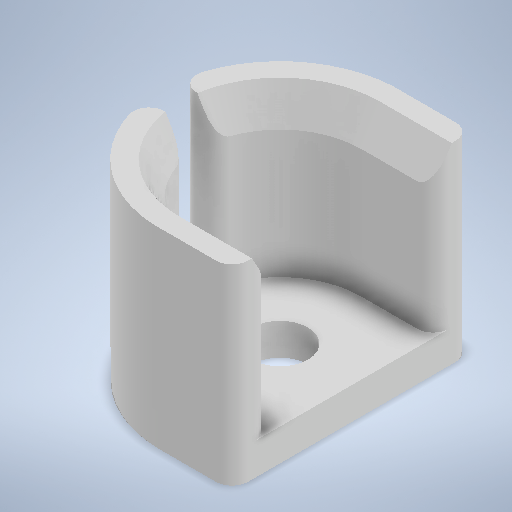
# Autodesk Inventor part: Align_Bracket
Saved by Autodesk Inventor 2025.1 (Build 291241000, 241)
## iProperties
Created: 2026-04-27
Part Number: Align_Bracket
Material: Generic
Document SubType Name: Modeling
Designer: ryand
Density: 1 g/cm^3
Appearance: Default
Author: ryand
Autodesk Inventor part; units mm, degrees
ref_plane "YZ Plane" through (0, 0, 0) normal (1, 0, 0) x (0, 1, 0)
ref_plane "XZ Plane" through (0, 0, 0) normal (0, 1, 0) x (-1, 0, 0)
ref_plane "XY Plane" through (0, 0, 0) normal (0, 0, 1) x (1, 0, 0)
sketch "Sketch1" plane through (0, 0, 0) normal (0, 1, 0) x (-1, 0, 0)
  line L0 (0, 7.5) -> (4.5, 7.5)
  line L1 (4.5, -7.5) -> (0, -7.5)
  line L2 (0, -7.5) -> (0, 7.5)
  arc A0 (4.5, -7.5) -> (4.5, 7.5) centre (4.5, 0) ccw
  point P0 (0, 0)
  point P1 (2.25, 7.5)
  dimension "d3" = 15
  dimension "d4" = 4.5
  dimension "d5" = 7.5
  dimension "d6" = 15
  constraints: 6 end point, 2 point on circle, 1 centre point, 1 horizontal, 1 midpoint, 1 parallel
  measures "d3" distance of L1.end L0.start
  measures "d4" distance of L0.start L0.end
  measures "d5" radius of A0
  measures "d6" distance of L1.start L0.end
extrude "Extrusion1" add sketch "Sketch1" along normal blind 2
sketch "Sketch2" plane through (0, 2, 0) normal (0, 1, 0) x (1, 0, 0)
  line L0 (0, -5.1) -> (-4.5, -5.1)
  line L1 (-4.5, -5.1) -> (-4.5, 5.1)
  line L2 (-4.5, 5.1) -> (0, 5.1)
  line L3 (0, 5.1) -> (0, -5.1)
  line L4 (0, -7.5) -> (0, 7.5) projected
  arc A0 (-4.5, 5.1) -> (-4.5, -5.1) centre (-4.5, 0) ccw
  line L5 (-5, -7.5) -> (0, -7.5)
  line L6 (0, 7.5) -> (-5, 7.5)
  arc A1 (-5, 7.5) -> (-5, -7.5) centre (-4.5, 0) ccw
  point P0 (0, 0)
  point P1 (0, 0)
  dimension "d9" = 4.5
  dimension "d10" = 10.2
  dimension "d11" = 5.1
  dimension "d30" = 5
  constraints: 12 end point, 4 point on circle, 3 horizontal, 2 centre point, 2 midpoint, 2 parallel, 1 coincident, 1 perpendicular
  measures "d9" distance of L1.end L2.end
  measures "d10" distance of L0.end L1.end
  measures "d11" distance of point (0, 0) L0.start
  measures "d30" distance of L5.start L4.start
extrude "Extrusion2" add sketch "Sketch2" along normal blind 10 contours L4 L5 A1 L6 L2 A0 L0
sketch "Sketch3" plane through (0, 12, 0) normal (0, 1, 0) x (1, 0, 0)
  line L0 (-13, -1) -> (-9, -1)
  line L1 (-9, -1) -> (-9, 1)
  line L2 (-9, 1) -> (-13, 1)
  line L3 (-13, 1) -> (-13, -1)
  line L4 (0, -5.1) -> (0, 5.1) projected
  point P0 (0, 0)
  dimension "d14" = 4
  dimension "d15" = 2
  dimension "d16" = 1
  dimension "d31" = 9
  constraints: 8 end point, 2 parallel, 1 horizontal, 1 perpendicular
  measures "d14" distance of L2.end L1.end
  measures "d15" distance of L1.end L0.end
  measures "d16" distance from line of point (0, 0) L0
  measures "d31" distance between parallel lines of L4 L1
extrude "Extrusion3" cut sketch "Sketch3" against normal blind 10
sketch "Sketch4" plane through (0, 2, 0) normal (0, 1, 0) x (1, 0, 0)
  circle A0 centre (-4.5, 0) radius 1.75
  line L0 (0, -5.1) -> (0, 5.1) projected
  point P0 (0, 0)
  point P1 (0, 0)
  dimension "d19" = 3.5
  dimension "d20" = 4.5
  constraints: 1 centre point, 1 midpoint
  measures "d19" diameter of A0
  measures "d20" distance of point (0, 0) A0.centre
extrude "Extrusion4" cut sketch "Sketch4" against normal blind 2
chamfer "Chamfer1" distance 2 angle 30 2 edges at (-2.25, 12, 5.1) (-7.7334, 12, 3.944) measured on face at (-7.7334, 11.5, 3.944) measured on face at (-2.25, 11.5, 5.1)
chamfer "Chamfer2" distance 2 angle 30 2 edges at (-2.25, 12, -5.1) (-7.7334, 12, -3.944) measured on face at (-2.25, 11.5, -5.1) measured on face at (-7.7334, 11.5, -3.944)
fillet "Fillet1" radius 1 6 edges at (-9.501, 6, 1) (-9.501, 6, -1) (0, 6, 7.5) (0, 6, 5.1) (0, 6, -5.1) (0, 6, -7.5)
fillet "Fillet2" radius 1 2 edges at (-11.9498, 7, -1) (-11.9498, 7, 1)
body "Solid1"
